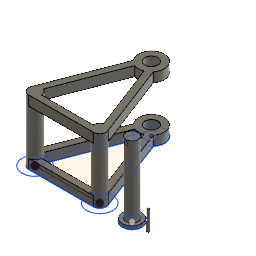
filament_holder v3 (Autodesk Fusion 360 design; units mm, degrees)
Autodesk Fusion 360 part; units mm, degrees
sketch "Sketch1" plane through (0, 0, 0) normal (0, 1, 0) x (1, 0, 0)
  line L0 (0, 0) -> (100, 0)
  line L1 (50, 130) -> (0, 0)
  line L2 (50, 130) -> (100, 0)
  circle A0 centre (100, 0) radius 9.9475
  circle A1 centre (50, 130) radius 10
  circle A2 centre (0, 0) radius 9.9475
  circle A3 centre (100, 0) radius 20
  circle A4 centre (0, 0) radius 20
  circle A5 centre (50, 130) radius 20
  line L3 (0, -9.9475) -> (100, -9.9475)
  line L4 (109.4834, 3.0031) -> (59.3353, 133.5851)
  line L5 (-9.0543, 4.1198) -> (40.6647, 133.5851)
  dimension "d8" = 100
  measures "d8" distance of L0.start
extrude "Extrude1" add sketch "Sketch1" along normal blind 15 contours L0 L1 A2 | L0 A2 A4 L3 | L1 A2 A4 L5 | L0 A3 A4 L3 | L1 A4 A5 L5 | L0 A0 A3 L3 | L1 A1 A5 L5 | L1 L2 A1 A5 | L0 L2 A0 L4 | L2 A0 A3 L4 | L2 A3 A5 L4 | A1 A5 L4 L5 | L2 A1 A5 L4 | A0 L4 picked at (6.5979, -0.4719) makes body 1
extrude "Extrude2" add sketch "Sketch1" along normal blind 100 contours L0 L1 A2 | L0 L1 A2 | L0 L2 A0 | L0 L2 A0 L4 | A0 L4 bodies 1
extrude "Extrude3" add sketch "Sketch1" against normal blind 15 from surface at 100 contours L0 L1 A2 | L0 L1 A2 | L0 A2 A4 L3 | L1 A2 A4 L5 | L0 A3 A4 L3 | L1 A4 A5 L5 | L0 A0 A3 L3 | L1 A1 A5 L5 | L1 L2 A1 A5 | L0 L2 A0 | L0 L2 A0 L4 | L2 A0 A3 L4 | L2 A3 A5 L4 | A1 A5 L4 L5 | L2 A1 A5 L4 | A0 L4 bodies 1
sketch "Sketch2" plane through (0, 0, 0) normal (0, 1, 0) x (1, 0, 0)
  circle A0 centre (150, 0) radius 9.5
  circle A1 centre (150, 0) radius 15
  dimension "d9" = 19
  measures "d9" diameter of A0
extrude "Extrude4" add sketch "Sketch2" along normal blind 115 separate body contours A0 makes body 2
extrude "Extrude5" add sketch "Sketch2" along normal blind 5 bodies 2
sketch "Sketch3" plane through (0, 0, 0) normal (0, 0, 1) x (1, 0, 0)
  circle A0 centre (150, 110) radius 2.5
  dimension "d14" = 5
  measures "d14" diameter of A0
extrude "Extrude6" cut sketch "Sketch3" along normal mid plane 40 bodies 2
sketch "Sketch4" plane through (0, 0, 0) normal (0, 1, 0) x (1, 0, 0)
  circle A0 centre (175, 0) radius 2.5
  dimension "d17" = 5
  measures "d17" diameter of A0
extrude "Extrude7" add sketch "Sketch4" along normal blind 30 draft -1 separate body makes body 3
